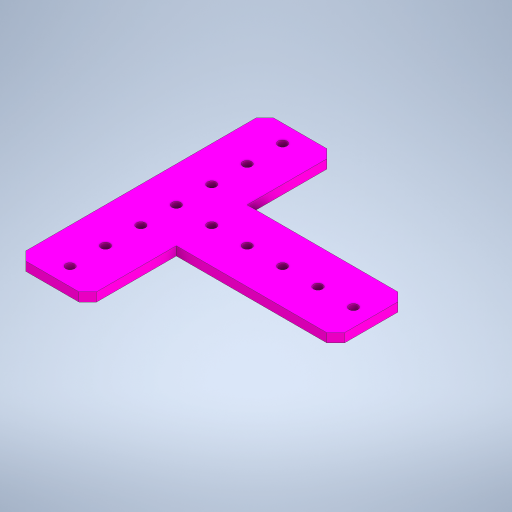
# Autodesk Inventor part: T-Bracket
Saved by Autodesk Inventor 2023 (Build 270158030, 158C)
## iProperties
Created: 2022-07-21
Part Number: T-Bracket
Material: Generic
Document SubType Name: Modeling
Designer: rm0990889
Density: 1 g/cm^3
Appearance: Default
Author: rm0990889
Autodesk Inventor part; units mm, degrees
ref_plane "YZ Plane" through (0, 0, 0) normal (1, 0, 0) x (0, 1, 0)
ref_plane "XZ Plane" through (0, 0, 0) normal (0, 1, 0) x (-1, 0, 0)
ref_plane "XY Plane" through (0, 0, 0) normal (0, 0, 1) x (1, 0, 0)
sketch "Sketch1" plane through (0, 0, 0) normal (0, 1, 0) x (-1, 0, 0)
  line L0 (9.8554, 3.698) -> (9.8554, -5.5599)
  line L1 (0, 0) -> (-5.6892, 0)
  circle A0 centre (-2.8446, 0) radius 1.5875
  circle A1 centre (-2.8446, -12.7) radius 1.5875
  circle A2 centre (-2.8446, -25.4) radius 1.5875
  circle A3 centre (-2.8446, -38.1) radius 1.5875
  line L2 (0, 12.7) -> (-5.6892, 12.7)
  circle A4 centre (-2.8446, 12.7) radius 1.5875
  line L3 (0, 25.4) -> (-5.6892, 25.4)
  circle A5 centre (-2.8446, 25.4) radius 1.5875
  line L4 (0, 38.1) -> (-5.6892, 38.1)
  circle A6 centre (-2.8446, 38.1) radius 1.5875
  line L5 (-12.7, 0) -> (-18.3892, 0)
  circle A7 centre (-15.5446, 0) radius 1.5875
  line L6 (-25.4, 0) -> (-31.0892, 0)
  circle A8 centre (-28.2446, 0) radius 1.5875
  line L7 (-38.1, 0) -> (-43.7892, 0)
  circle A9 centre (-40.9446, 0) radius 1.5875
  line L8 (-50.8, 0) -> (-56.4892, 0)
  circle A10 centre (-53.6446, 0) radius 1.5875
  line L9 (-63.5, 0) -> (-69.1892, 0)
  circle A11 centre (-66.3446, 0) radius 1.5875
  line L10 (9.8554, 3.698) -> (9.8554, 44.45)
  line L11 (9.8554, 44.45) -> (-15.5446, 44.45)
  line L12 (-15.5446, 44.45) -> (-15.5446, 12.7)
  line L13 (-15.5446, 12.7) -> (-72.6946, 12.7)
  line L14 (-72.6946, 12.7) -> (-72.6946, -12.7)
  line L15 (-72.6946, -12.7) -> (-15.5446, -12.7)
  line L16 (-15.5446, -12.7) -> (-15.5446, -44.45)
  line L17 (-15.5446, -44.45) -> (9.8554, -44.45)
  line L18 (9.8554, -5.5599) -> (9.8554, -44.45)
  line L19 (-12.3696, 44.45) -> (-15.5446, 41.275)
  line L20 (6.6804, 44.45) -> (9.8554, 41.275)
  line L21 (9.8554, -41.275) -> (6.6804, -44.45)
  line L22 (-15.5446, -41.275) -> (-12.3696, -44.45)
  line L23 (-69.5196, 12.7) -> (-72.6946, 9.525)
  line L24 (-72.6946, -9.525) -> (-69.5196, -12.7)
  point P0 (-72.6946, 0)
  point P1 (-66.3446, 0)
  dimension "d0" = 3.175
  dimension "d1" = 12.7
  dimension "d4" = 12.7
  dimension "d11" = 12.7
  dimension "d18" = 12.7
  dimension "d23" = 25.4
  dimension "d24" = 6.35
  dimension "d25" = 12.7
  dimension "d26" = 6.35
  dimension "d27" = 25.4
  constraints: 50 end point, 12 centre point, 12 point on line, 7 vertical, 5 midpoint, 4 perpendicular, 3 equal length, 3 horizontal, 1 collinear, 45 other
  measures "d0" diameter of A0
  measures "d1" distance from line of A0.centre L0
  measures "d4" distance of A0.centre A1.centre
  measures "d11" distance of L1.end L2.end
  measures "d18" distance of L1.end L5.end
  measures "d23" distance of L10.end L11.end
  measures "d24" distance from line of point (-2.845, 38.1) L11
  measures "d25" distance of point (-15.545, 0) L12.end
  measures "d26" distance of point (-72.695, 0) point (-66.345, 0)
  measures "d27" distance of L13.end L14.end
extrude "Extrusion1" add sketch "Sketch1" along normal blind 3.175 contours L0 L18 L21 L17 L22 L16 L15 L24 L14 L23 L13 L12 L19 L11 L20 L10
body "Solid1"
